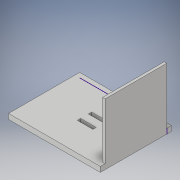
# Autodesk Inventor part: Boxpt2
Saved by Autodesk Inventor 2018.2 (Build 222227000, 227)
## iProperties
Created: 2018-04-06
Part Number: Boxpt2
Material: Generic
Document SubType Name: Modeling
Designer: MIABo
Density: 1 g/cm^3
Appearance: Default
Author: MIABo
## iProperties of the stored document Boxpt2_3DPrint.ipt
Created: 2018-04-09
Part Number: Boxpt2_3DPrint
Material: Generic
Document SubType Name: Modeling
Designer: MIABo
Density: 1 g/cm^3
Appearance: Default
Author: MIABo
Autodesk Inventor part; units mm, degrees
ref_plane "YZ Plane" through (0, 0, 0) normal (1, 0, 0) x (0, 1, 0)
ref_plane "XZ Plane" through (0, 0, 0) normal (0, 1, 0) x (-1, 0, 0)
ref_plane "XY Plane" through (0, 0, 0) normal (0, 0, 1) x (1, 0, 0)
sketch "Sketch1" plane through (0, 0, 0) normal (0, 1, 0) x (-1, 0, 0)
  line L0 (53.2003, -37.719) -> (-53.2003, -37.719)
  line L1 (-53.2003, -37.719) -> (-53.2003, 37.719)
  line L2 (-53.2003, 37.719) -> (53.2003, 37.719)
  line L3 (53.2003, 37.719) -> (53.2003, -37.719)
  line L4 (53.2003, -37.719) -> (-53.2003, 37.719) construction
  line L5 (-53.2003, -37.719) -> (53.2003, 37.719) construction
  point P0 (0, 0)
  dimension "d0" = 106.4006
  dimension "d1" = 75.438
  constraints: 12 end point, 2 midpoint, 2 parallel, 1 horizontal, 1 perpendicular
  measures "d0" distance of L1.end L2.end
  measures "d1" distance of L0.end L1.end
extrude "Extrusion1" add sketch "Sketch1" along normal blind 6.35
sketch "Sketch2" plane through (0, 6.35, 0) normal (0, 1, 0) x (1, 0, 0)
  line L0 (53.2003, -37.719) -> (53.2003, 37.719) projected
  line L1 (53.2003, -37.719) -> (53.2003, -34.544)
  line L2 (53.2003, -34.544) -> (50.0761, -34.544)
  line L3 (53.2003, 37.719) -> (53.2003, 34.544)
  line L4 (53.2003, 34.544) -> (50.0761, 34.544)
  line L5 (50.0761, 34.544) -> (50.0761, -34.544)
  line L6 (53.2003, -34.544) -> (53.2003, 34.544)
  point P0 (0, 0)
  dimension "d4" = 3.175
  dimension "d5" = 3.1242
  dimension "d6" = 3.175
  constraints: 12 end point, 3 perpendicular, 2 point on line, 1 collinear
  measures "d4" distance of L0.start L1.end
  measures "d5" distance of L1.end L2.end
  measures "d6" distance of L0.end L3.end
extrude "Extrusion2" add sketch "Sketch2" along normal blind 68.58
fillet "Fillet1" radius 3.175 1 edges at (50.0761, 6.35, 0)
sketch "Sketch3" plane through (0, 0, 0) normal (0, -1, 0) x (1, 0, 0)
  line L0 (-9.525, 8.763) -> (9.525, 8.763)
  line L1 (9.525, 8.763) -> (9.525, -8.763)
  line L2 (9.525, -8.763) -> (-9.525, -8.763)
  line L3 (-9.525, -8.763) -> (-9.525, 8.763)
  line L4 (-9.525, 8.763) -> (9.525, -8.763) construction
  line L5 (9.525, 8.763) -> (-9.525, -8.763) construction
  line L6 (9.525, -8.763) -> (-9.525, -8.763)
  line L7 (-9.525, -8.763) -> (-9.525, -4.699)
  line L8 (-9.525, -4.699) -> (9.525, -4.699)
  line L9 (9.525, -4.699) -> (9.525, -8.763)
  line L10 (9.525, 8.763) -> (-9.525, 8.763)
  line L11 (-9.525, 8.763) -> (-9.525, 4.699)
  line L12 (-9.525, 4.699) -> (9.525, 4.699)
  line L13 (9.525, 4.699) -> (9.525, 8.763)
  point P0 (0, 0)
  dimension "d10" = 19.05
  dimension "d11" = 17.526
  dimension "d12" = 4.064
  dimension "d13" = 4.064
  constraints: 28 end point, 6 parallel, 3 horizontal, 3 perpendicular, 2 midpoint, 2 point on line
  measures "d10" distance of L1.end L2.end
  measures "d11" distance of L0.end L1.end
  measures "d12" distance of L6.end L7.end
  measures "d13" distance of L11.end L10.end
extrude "Extrusion3" cut sketch "Sketch3" against normal blind 68.58 contours L0 L1 L12 L3 | L8 L1 L2 L3
sketch "Sketch4" plane through (0, 0, 0) normal (0, -1, 0) x (1, 0, 0)
  point P0 (0, 0)
sketch "Sketch5" plane through (0, 0, 0) normal (0, -1, 0) x (1, 0, 0)
  point P0 (0, 0)
sketch "Sketch6" plane through (53.2003, 0, -37.719) normal (0, 0, -1) x (-1, 0, 0)
  line L0 (106.4006, 0) -> (0, 0) projected
  line L1 (0, 6.35) -> (106.4006, 6.35) projected
  line L2 (106.4006, 0) -> (0, 0)
  line L3 (0, 0) -> (0, 6.35)
  line L4 (0, 6.35) -> (106.4006, 6.35)
  line L5 (106.4006, 6.35) -> (106.4006, 0)
  point P0 (53.2003, 0)
  constraints: 8 end point, 2 parallel, 1 horizontal, 1 perpendicular
sketch "Sketch7" plane through (0, 6.35, 0) normal (0, 1, 0) x (1, 0, 0)
  line L0 (53.2003, 34.544) -> (53.2003, 37.719) projected
  line L1 (46.9519, -37.719) -> (53.2003, -37.719)
  line L2 (53.2003, -37.719) -> (53.2003, 37.719)
  line L3 (53.2003, 37.719) -> (46.9519, 37.719)
  line L4 (46.9519, 37.719) -> (46.9519, -37.719)
  line L5 (50.0761, 34.544) -> (50.0761, -34.544) projected
  line L6 (46.9519, -37.719) -> (53.2003, 37.719) construction
  line L7 (53.2003, -37.719) -> (46.9519, 37.719) construction
  point P0 (0, 0)
  point P1 (50.0761, 0)
  constraints: 12 end point, 3 midpoint, 2 parallel, 1 horizontal, 1 perpendicular
extrude "Extrusion4" add sketch "Sketch7" along normal blind 68.58
sketch "Sketch8" plane through (0, 74.93, 0) normal (0, 1, 0) x (1, 0, 0)
  line L0 (53.2003, -37.719) -> (53.2003, 37.719) projected
  line L1 (53.2003, 37.719) -> (46.9519, 37.719) projected
  line L2 (53.2003, -37.719) -> (50.0761, -37.719)
  line L3 (50.0761, -37.719) -> (50.0761, 37.719)
  line L4 (50.0761, 37.719) -> (53.2003, 37.719)
  line L5 (53.2003, 37.719) -> (53.2003, -37.719)
  line L6 (46.9519, -37.719) -> (53.2003, -37.719) projected
  line L7 (50.0761, 37.719) -> (46.9519, 37.719)
  line L8 (46.9519, 37.719) -> (46.9519, -37.719)
  line L9 (46.9519, -37.719) -> (50.0761, -37.719)
  line L10 (50.0761, -37.719) -> (50.0761, 37.719)
  point P0 (0, 0)
  constraints: 16 end point, 4 parallel, 2 horizontal, 2 perpendicular, 1 midpoint
extrude "Extrusion5" cut sketch "Sketch8" against normal blind 68.58 contours L6 L8 L1 L3
sketch "Sketch9" plane through (53.2003, 0, -37.719) normal (0, 0, -1) x (-1, 0, 0)
  line L0 (3.1242, 6.35) -> (106.4006, 6.35) projected
  line L1 (106.4006, 6.35) -> (0, 6.35)
  line L2 (0, 6.35) -> (0, 0)
  line L3 (0, 0) -> (106.4006, 0)
  line L4 (106.4006, 0) -> (106.4006, 6.35)
  point P0 (53.2003, 0)
  constraints: 8 end point, 2 parallel, 1 horizontal, 1 perpendicular
extrude "Extrusion6" add sketch "Sketch9" along normal blind 5.715
sketch "Sketch10" plane through (-53.2003, 0, 37.719) normal (0, 0, 1) x (1, 0, 0)
  line L0 (0, 6.35) -> (106.4006, 6.35) projected
  line L1 (106.4006, 0) -> (106.4006, 74.93) projected
  line L2 (0, 6.35) -> (106.4006, 6.35)
  line L3 (106.4006, 6.35) -> (106.4006, 0)
  line L4 (106.4006, 0) -> (0, 0)
  line L5 (0, 0) -> (0, 6.35)
  point P0 (53.2003, 0)
  constraints: 8 end point, 2 parallel, 1 horizontal, 1 perpendicular
extrude "Extrusion7" add sketch "Sketch10" along normal blind 5.715
sketch "Sketch11" plane through (-53.2003, 0, -43.434) normal (-1, 0, 0) x (0, 0, 1)
  line L0 (0, 0) -> (0, 6.35) projected
  line L1 (86.868, 0) -> (0, 0) projected
  line L2 (0, 6.35) -> (86.868, 6.35)
  line L3 (86.868, 6.35) -> (86.868, 0)
  line L4 (86.868, 0) -> (0, 0)
  line L5 (0, 0) -> (0, 6.35)
  point P0 (43.434, 0)
  constraints: 8 end point, 2 parallel, 1 horizontal, 1 perpendicular
extrude "Extrusion8" add sketch "Sketch11" along normal blind 5.715
body "Solid1"
